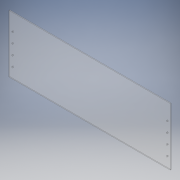
# Autodesk Inventor part: LexanSheetCoverForIntake
Saved by Autodesk Inventor 2018.3 (Build 223284000, 284)
## iProperties
Created: 2020-02-14
Part Number: LexanSheetCoverForIntake
Material: Polycarbonate, Clear
Document SubType Name: Modeling
Designer: 22oktynich
Density: 1.2 g/cm^3
Appearance: Polycarbonate - Clear
Author: 22oktynich
Autodesk Inventor part; units mm, degrees
ref_plane "YZ Plane" through (0, 0, 0) normal (1, 0, 0) x (0, 1, 0)
ref_plane "XZ Plane" through (0, 0, 0) normal (0, 1, 0) x (-1, 0, 0)
ref_plane "XY Plane" through (0, 0, 0) normal (0, 0, 1) x (1, 0, 0)
sketch "Sketch1" plane through (0, 0, 0) normal (0, 0, 1) x (1, 0, 0)
  line L0 (0, 0) -> (-603.25, 0)
  line L1 (-603.25, 0) -> (-603.25, 215.9)
  line L2 (-603.25, 215.9) -> (0, 215.9)
  line L3 (0, 215.9) -> (0, 0)
  dimension "d0" = 603.25
  dimension "d1" = 215.9
  constraints: 8 end point, 2 parallel, 1 horizontal, 1 perpendicular
  measures "d0" distance of L1.end L2.end
  measures "d1" distance of L2.end L0.start
extrude "Extrusion1" add sketch "Sketch1" along normal blind 3.175
sketch "Sketch2" plane through (0, 0, 3.175) normal (0, 0, 1) x (1, 0, 0)
  line L0 (0, 215.9) -> (-603.25, 215.9) projected
  line L1 (-603.25, 0) -> (0, 0) projected
  line L2 (0, 0) -> (0, 215.9) projected
  line L3 (-301.625, 215.9) -> (-301.625, 0)
  line L4 (-603.25, 215.9) -> (-603.25, 0) projected
  point P0 (-12.7, 38.1)
  point P1 (-12.7, 76.2)
  point P2 (-12.7, 114.3)
  point P3 (-12.7, 152.4)
  point P4 (-590.55, 38.1)
  point P5 (-590.55, 76.2)
  point P6 (-590.55, 114.3)
  point P7 (-590.55, 152.4)
  dimension "d8" = 38.1
  dimension "d9" = 38.1
  dimension "d10" = 38.1
  dimension "d11" = 63.5
  dimension "d12" = 12.7
  dimension "d13" = 301.625
  constraints: 4 symmetric about line, 3 vertical alignment, 2 end point, 2 midpoint, 1 vertical
  measures "d8" distance of point (-12.7, 114.3) point (-12.7, 152.4)
  measures "d9" distance of point (-12.7, 76.2) point (-12.7, 114.3)
  measures "d10" distance of point (-12.7, 38.1) point (-12.7, 76.2)
  measures "d11" distance from line of L0 point (-12.7, 152.4)
  measures "d12" distance from line of L2 point (-12.7, 152.4)
  measures "d13" distance between parallel lines of L4 L3
hole "Hole1" at (-12.7, 38.1, 3.175) at (-12.7, 76.2, 3.175) at (-12.7, 114.3, 3.175) at (-12.7, 152.4, 3.175) at (-590.55, 152.4, 3.175) at (-590.55, 114.3, 3.175) at (-590.55, 76.2, 3.175) at (-590.55, 38.1, 3.175) direction (0, 0, -1) diameter 4.8514 end through all
body "Solid1"
